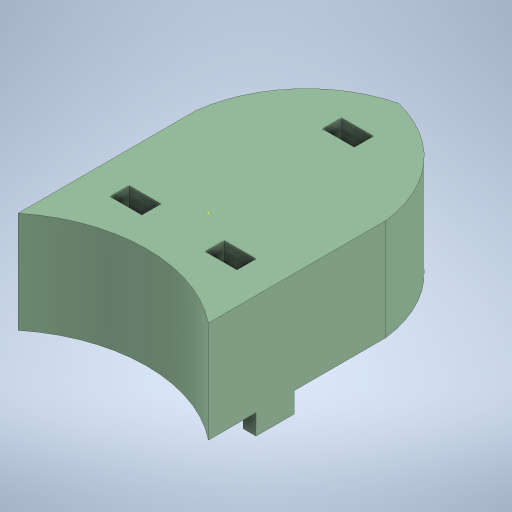
# Autodesk Inventor part: NORGATE
Saved by Autodesk Inventor 2024 (Build 280153000, 153)
## iProperties
Created: 2024-01-22
Part Number: NORGATE
Material: Generic
Document SubType Name: Modeling
Designer: Jetsan
Density: 1 g/cm^3
Appearance: Rubber - Green
Author: Jetsan
Autodesk Inventor part; units mm, degrees
ref_plane "YZ Plane" through (0, 0, 0) normal (1, 0, 0) x (0, 1, 0)
ref_plane "XZ Plane" through (0, 0, 0) normal (0, 1, 0) x (-1, 0, 0)
ref_plane "XY Plane" through (0, 0, 0) normal (0, 0, 1) x (1, 0, 0)
sketch "Sketch1" plane through (0, 0, 0) normal (0, 1, 0) x (-1, 0, 0)
  line L0 (-7.5, 7.5) -> (7.5, 7.5)
  line L1 (7.5, 7.5) -> (7.5, -7.5)
  line L2 (7.5, -7.5) -> (-7.5, -7.5)
  line L3 (-7.5, -7.5) -> (-7.5, 7.5)
  line L4 (-7.5, 7.5) -> (7.5, -7.5) construction
  line L5 (7.5, 7.5) -> (-7.5, -7.5) construction
  circle A0 centre (0, -7.5) radius 7.5 construction
  arc A1 (-7.5, -7.5) -> (7.5, -7.5) centre (0, -7.5) ccw
  arc A2 (0, -15) -> (7.5, -6.5) centre (-2.4276, -5.2991) ccw
  arc A3 (-7.5, -6.5) -> (0, -15) centre (2.4276, -5.2991) ccw
  point P0 (0, 0)
  dimension "d0" = 15
  dimension "d1" = 15
  dimension "d106" = 10
  dimension "d107" = 10
  dimension "d108" = 14
  dimension "d109" = 14
  constraints: 12 end point, 7 point on circle, 3 centre point, 3 midpoint, 2 parallel, 2 point on line, 1 coincident, 1 horizontal, 1 horizontal alignment, 1 perpendicular, 2 other
  measures "d0" distance of L0.end L1.end
  measures "d1" distance of L0.start L0.end
  measures "d106" radius of A2
  measures "d107" radius of A3
  measures "d108" distance from line of L0 A2.end
  measures "d109" distance from line of L0 A3.start
extrude "Extrusion1" add sketch "Sketch1" along normal blind 8 contours L0 L1 A2 L2 A3 L3 | L2 A2 A3
sketch "Sketch2" plane through (0, 0, 0) normal (0, -1, 0) x (1, 0, 0)
  line L0 (7.5, 11.25) -> (-7.5, 11.25)
  line L1 (-7.5, 11.25) -> (-7.5, -18.75)
  line L2 (-7.5, -18.75) -> (7.5, -18.75)
  line L3 (7.5, -18.75) -> (7.5, 11.25)
  line L4 (7.5, 11.25) -> (-7.5, -18.75) construction
  line L5 (-7.5, 11.25) -> (7.5, -18.75) construction
  line L6 (-7.5, 7.5) -> (7.5, 7.5) projected
  line L7 (7, 10.75) -> (-7, 10.75) construction
  line L8 (-7, 10.75) -> (-7, -18.25) construction
  line L9 (-7, -18.25) -> (7, -18.25) construction
  line L10 (7, -18.25) -> (7, 10.75) construction
  line L11 (7, 10.75) -> (-7, -18.25) construction
  line L12 (-7, 10.75) -> (7, -18.25) construction
  arc A0 (-7.5, 11.25) -> (7.5, 11.25) centre (0, 17.8644) ccw
  point P0 (0, 0)
  point P1 (0, -3.75)
  dimension "d4" = 15
  dimension "d5" = 30
  dimension "d6" = 3.75
  dimension "d18" = 0.5
  dimension "d19" = 0.5
  dimension "d99" = 10
  constraints: 24 end point, 4 midpoint, 4 parallel, 2 horizontal, 2 perpendicular, 2 point on circle, 1 centre point
  measures "d4" distance of L2.end L1.end
  measures "d5" distance of L1.end L0.end
  measures "d6" distance between parallel lines of L0 L6
  measures "d18" distance between parallel lines of L2 L9
  measures "d19" distance between parallel lines of L3 L10
  measures "d99" radius of A0
sketch "Sketch4" plane through (0, 0, 0) normal (0, -1, 0) x (1, 0, 0)
  line L0 (-7.5, -6.5) -> (-7.5, 7.5) projected
  line L1 (-7.5, 3.75) -> (-6.5, 3.75)
  line L2 (-6.5, 3.75) -> (-6.5, 0.75)
  line L3 (-6.5, 0.75) -> (-7.5, 0.75)
  line L4 (-7.5, 0.75) -> (-7.5, 3.75)
  line L5 (7.5, 7.5) -> (7.5, -6.5) projected
  line L6 (7.5, 0.75) -> (6.5, 0.75)
  line L7 (6.5, 0.75) -> (6.5, 3.75)
  line L8 (6.5, 3.75) -> (7.5, 3.75)
  line L9 (7.5, 3.75) -> (7.5, 0.75)
  line L10 (-7.5, -18.75) -> (7.5, -18.75) construction
  line L11 (7.5, -18.75) -> (7.5, 11.25) construction
  line L12 (7.5, 11.25) -> (-7.5, 11.25) construction
  line L13 (-7.5, 11.25) -> (-7.5, -18.75) construction
  line L14 (-7.5, -18.75) -> (7.5, 11.25) construction
  line L15 (7.5, -18.75) -> (-7.5, 11.25) construction
  line L16 (-7.5, 7.5) -> (7.5, 7.5) construction
  arc A0 (-7.5, -7.5) -> (7.5, -7.5) centre (0, -7.5) ccw construction
  point P0 (0, 0)
  point P1 (0, -3.75)
  point P2 (0, -15)
  point P3 (-7, 3.75)
  point P4 (7.5, 3.75)
  dimension "d20" = 1
  dimension "d21" = 3
  dimension "d22" = 1
  dimension "d23" = 3
  dimension "d24" = 15
  dimension "d25" = 30
  dimension "d26" = 3.75
  dimension "d27" = 3.75
  dimension "d28" = 7.5
  constraints: 28 end point, 6 parallel, 3 horizontal, 3 midpoint, 3 perpendicular, 3 point on line, 1 point on circle
  measures "d20" distance of L2.end L3.end
  measures "d21" distance of L1.end L2.end
  measures "d22" distance of L7.end L8.end
  measures "d23" distance of L6.end L7.end
  measures "d24" distance of L12.end L11.end
  measures "d25" distance of L11.end L10.end
  measures "d26" distance between parallel lines of L16 L12
  measures "d27" distance from line of L10 point (0, -15)
  measures "d28" distance from line of L12 point (-7, 3.75)
extrude "Extrusion3" add sketch "Sketch4" along normal blind 1.6
sketch "Sketch17" plane through (0, 0, 0) normal (0, -1, 0) x (1, 0, 0)
  line L0 (-7.5, 7.5) -> (7.5, 7.5) projected
  arc A0 (-7.5, 7.5) -> (7.5, 7.5) centre (0, 16.8675) ccw
  line L1 (7.5, 7.5) -> (-7.5, 7.5)
  point P0 (0, 0)
  dimension "d100" = 12
  constraints: 2 end point, 2 point on circle, 1 centre point, 1 horizontal
  measures "d100" radius of A0
extrude "Extrusion11" cut sketch "Sketch17" against normal blind 8
sketch "Sketch6" plane through (0, 0, 0) normal (0, -1, 0) x (1, 0, 0)
  line L0 (7.5, 11.25) -> (-7.5, 11.25)
  line L1 (-7.5, 11.25) -> (-7.5, -18.75)
  line L2 (-7.5, -18.75) -> (7.5, -18.75)
  line L3 (7.5, -18.75) -> (7.5, 11.25)
  line L4 (7.5, 11.25) -> (-7.5, -18.75) construction
  line L5 (-7.5, 11.25) -> (7.5, -18.75) construction
  line L6 (7, 10.75) -> (-7, 10.75) construction
  line L7 (-7, 10.75) -> (-7, -18.25) construction
  line L8 (-7, -18.25) -> (7, -18.25) construction
  line L9 (7, -18.25) -> (7, 10.75) construction
  line L10 (7, 10.75) -> (-7, -18.25) construction
  line L11 (-7, 10.75) -> (7, -18.25) construction
  circle A0 centre (0, -3.75) radius 1.25
  circle A1 centre (0, -3.75) radius 1.75
  line L12 (-6.5, 6.5) -> (6.5, 6.5)
  line L13 (6.5, 6.5) -> (6.5, -7.5)
  line L14 (6.5, -7.5) -> (-6.5, -7.5)
  line L15 (-6.5, -7.5) -> (-6.5, 6.5)
  line L16 (-7.5, 7.5) -> (7.5, 7.5) projected
  arc A2 (-7.5, -7.5) -> (7.5, -7.5) centre (0, -7.5) ccw projected
  circle A3 centre (0, -7.5) radius 6.5
  line L17 (0, 11.25) -> (0, -15) construction
  arc A4 (-6.5, 5.5) -> (6.5, 5.5) centre (0, 15.8675) ccw
  line L18 (6.5, 5.5) -> (-6.5, 5.5) construction
  line L19 (6.5, 5.5) -> (19.5, 5.5) construction
  arc A5 (-7.5, 7.5) -> (7.5, 7.5) centre (0, 16.8675) ccw projected
  point P0 (0, 0)
  point P1 (-7.5, -3.75)
  dimension "d31" = 15
  dimension "d32" = 30
  dimension "d34" = 0.5
  dimension "d35" = 0.5
  dimension "d36" = 2.5
  dimension "d37" = 0.5
  dimension "d38" = 1
  dimension "d39" = 1
  dimension "d40" = 1
  dimension "d41" = 1
  dimension "d103" = 180
  dimension "d104" = 1
  dimension "d105" = 1
  constraints: 38 end point, 6 midpoint, 6 parallel, 4 horizontal, 3 centre point, 3 coincident, 3 perpendicular, 3 point on circle, 2 point on line, 1 collinear, 3 other
  measures "d31" distance of L2.end L1.end
  measures "d32" distance of L1.end L0.end
  measures "d34" distance between parallel lines of L2 L8
  measures "d35" distance between parallel lines of L3 L9
  measures "d36" diameter of A0
  measures "d37" radial gap between concentric circles of A0 A1
  measures "d38" distance between parallel lines of L16 L12
  measures "d39" distance from line of point (-7.5, -3.75) L15
  measures "d40" distance between parallel lines of L3 L13
  measures "d103" angle of L18 L19
  measures "d104" distance of A5.centre A4.centre
  measures "d105" distance of L12.end L18.start
extrude "Extrusion4" cut sketch "Sketch6" against normal blind 2.5 contours L13 A3 L15 A4 | A3 L14 | L14 A3 | A0
sketch "Sketch10" plane through (0, 8, 0) normal (0, 1, 0) x (1, 0, 0)
  point P0 (0, 0)
sketch "Sketch11" plane through (0, 0, 0) normal (0, -1, 0) x (1, 0, 0)
  line L0 (-5, 2.75) -> (-2.5, 2.75)
  line L1 (-2.5, 2.75) -> (-2.5, 1.25)
  line L2 (-2.5, 1.25) -> (-5, 1.25)
  line L3 (-5, 1.25) -> (-5, 2.75)
  line L4 (2.5, 2.75) -> (5, 2.75)
  line L5 (5, 2.75) -> (5, 1.25)
  line L6 (5, 1.25) -> (2.5, 1.25)
  line L7 (2.5, 1.25) -> (2.5, 2.75)
  line L8 (-6.5, 3.75) -> (-7.5, 3.75) projected
  line L9 (-6.5, 0.75) -> (-6.5, 3.75) projected
  line L10 (6.5, 3.75) -> (6.5, 0.75) projected
  line L11 (-6.5, 6.5) -> (6.5, 6.5) projected
  line L12 (-1.25, -11.75) -> (1.25, -11.75)
  line L13 (1.25, -11.75) -> (1.25, -10.25)
  line L14 (1.25, -10.25) -> (-1.25, -10.25)
  line L15 (-1.25, -10.25) -> (-1.25, -11.75)
  point P0 (0, 0)
  point P1 (-3.75, 2.75)
  point P2 (3.75, 2.75)
  point P3 (1.25, -11)
  point P4 (2.5, 2)
  point P5 (0, -10.25)
  point P6 (3.75, 1.25)
  dimension "d51" = 2.5
  dimension "d52" = 1.5
  dimension "d53" = 1
  dimension "d55" = 2.75
  dimension "d56" = 2.75
  dimension "d57" = 3.75
  dimension "d60" = 13
  dimension "d61" = 3.75
  dimension "d62" = 3.75
  constraints: 24 end point, 6 midpoint, 6 parallel, 4 equal length, 3 horizontal, 3 perpendicular
  measures "d51" distance of L0.start L0.end
  measures "d52" distance of L0.end L1.end
  measures "d53" distance between parallel lines of L8 L0
  measures "d55" distance from line of L9 point (-3.75, 2.75)
  measures "d56" distance from line of L10 point (3.75, 2.75)
  measures "d57" distance between parallel lines of L11 L4
  measures "d60" vertical distance of point (1.25, -11) point (2.5, 2)
  measures "d61" horizontal distance of point (0, -10.25) point (3.75, 1.25)
  measures "d62" horizontal distance of point (0, -10.25) point (-3.75, 2.75)
extrude "Extrusion8" cut sketch "Sketch11" against normal blind 10
sketch "Sketch12" plane through (0, 2.5, 0) normal (0, -1, 0) x (1, 0, 0)
  line L0 (5, 1.25) -> (5, 2.75) construction
  line L1 (2.5, 1.25) -> (5, 1.25) construction
  line L2 (5, 2.75) -> (2.5, 2.75) construction
  line L3 (2.5, 2.75) -> (2.5, 1.25) construction
  line L4 (2.5, 1.25) -> (5, 1.25) construction
  line L5 (5, 1.25) -> (5, 2.75) construction
  line L6 (-2.5, 1.25) -> (-2.5, 2.75) construction
  line L7 (-2.5, 1.25) -> (-5, 1.25) construction
  line L8 (-2.5, 2.75) -> (-5, 2.75) construction
  line L9 (-5, 2.75) -> (-5, 1.25) construction
  line L10 (-5, 1.25) -> (-2.5, 1.25) construction
  line L11 (-2.5, 1.25) -> (-2.5, 2.75) construction
  line L12 (-1.25, -10.25) -> (1.25, -10.25) construction
  line L13 (-1.25, -10.25) -> (-1.25, -11.75) construction
  line L14 (1.25, -10.25) -> (-1.25, -10.25) construction
  line L15 (-1.25, -10.25) -> (-1.25, -11.75) construction
  line L16 (-1.25, -11.75) -> (1.25, -11.75) construction
  line L17 (1.25, -11.75) -> (1.25, -10.25) construction
  line L18 (5.5, 2.75) -> (2, 2.75)
  line L19 (2, 2.75) -> (2, 1.25)
  line L20 (2, 1.25) -> (5.5, 1.25)
  line L21 (5.5, 1.25) -> (5.5, 2.75)
  line L22 (1.75, -10.25) -> (-1.75, -10.25)
  line L23 (-1.75, -10.25) -> (-1.75, -11.75)
  line L24 (-1.75, -11.75) -> (1.75, -11.75)
  line L25 (1.75, -11.75) -> (1.75, -10.25)
  line L26 (-2, 2.75) -> (-5.5, 2.75)
  line L27 (-5.5, 2.75) -> (-5.5, 1.25)
  line L28 (-5.5, 1.25) -> (-2, 1.25)
  line L29 (-2, 1.25) -> (-2, 2.75)
  point P0 (0, 0)
  point P1 (-2.5, 2)
  point P2 (-2, 2)
  point P3 (-3.75, 1.25)
  point P4 (-3.75, 1.25)
  point P5 (-3.75, 2.75)
  point P6 (-3.75, 2.75)
  point P7 (-5, 2)
  point P8 (-5.5, 2)
  point P9 (1.25, -11)
  point P10 (1.75, -11)
  point P11 (0, -11.75)
  point P12 (-1.25, -11)
  dimension "d63" = 0.5
  dimension "d64" = 0
  dimension "d65" = 0
  dimension "d67" = 0.5
  dimension "d68" = 0
  dimension "d69" = 0
  dimension "d70" = 0.5
  dimension "d71" = 0.5
  dimension "d72" = 0
  dimension "d73" = 0
  dimension "d74" = 0.5
  dimension "d96" = 0.5
  constraints: 48 end point, 12 midpoint, 12 parallel, 6 horizontal, 6 perpendicular
  measures "d63" distance of point (-2.5, 2) point (-2, 2)
  measures "d64" distance of point (-3.75, 1.25) point (-3.75, 1.25)
  measures "d65" distance of point (-3.75, 2.75) point (-3.75, 2.75)
  measures "d67" distance of point (1.25, -11) point (1.75, -11)
  measures "d68" distance from line of L24 point (0, -11.75)
  measures "d69" distance between parallel lines of L22 L12
  measures "d70" distance from line of L23 point (-1.25, -11)
  measures "d71" distance between parallel lines of L0 L21
  measures "d72" distance between parallel lines of L20 L1
  measures "d73" distance between parallel lines of L18 L2
  measures "d74" distance between parallel lines of L19 L3
  measures "d96" distance between parallel lines of L27 L9
extrude "Extrusion9" cut sketch "Sketch12" against normal blind 1
sketch "Sketch16" plane through (0, 2.5, 0) normal (0, -1, 0) x (1, 0, 0)
  line L0 (-6.5, -7.5) -> (-6.5, 5.5) construction
  line L1 (-0.5, 4.8675) -> (0.5, 4.8675)
  line L2 (0.5, 4.8675) -> (0.5, -2.5)
  line L3 (0.5, -2.5) -> (-0.5, -2.5)
  line L4 (-0.5, -2.5) -> (-0.5, 4.8675)
  circle A0 centre (0, -3.75) radius 1.75 construction
  circle A1 centre (0, -3.75) radius 1.75 construction
  line L5 (-6.5, -2.5) -> (6.5174, -2.5) construction
  circle A2 centre (0, -3.75) radius 1.75 construction
  circle A3 centre (0, -3.75) radius 1.25 construction
  line L6 (6.5, 0.75) -> (6.5, -7.5) projected
  line L7 (-6.5, -5.873) -> (6.5, -5.873)
  line L8 (6.5, -5.873) -> (6.5, -6.873)
  line L9 (6.5, -6.873) -> (-6.5, -6.873)
  line L10 (-6.5, -6.873) -> (-6.5, -5.873)
  arc A4 (-7.5, 7.5) -> (7.5, 7.5) centre (0, 16.8675) ccw projected
  point P0 (0, 0)
  point P1 (-6.5, 6.5)
  point P2 (6.5, 6.5)
  point P3 (0, 4.8675)
  point P4 (0.0087, -2.5)
  dimension "d94" = 1
  dimension "d95" = 1
  constraints: 18 end point, 4 parallel, 4 point on line, 3 perpendicular, 2 horizontal, 2 midpoint, 1 centre point, 1 coincident, 1 point on circle, 1 tangent
  measures "d94" distance between parallel lines of L2 L4
  measures "d95" distance between parallel lines of L9 L7
extrude "Extrusion10" add sketch "Sketch16" along normal blind 2.5 contours L1 L2 L3 L4
sketch "Sketch14" plane through (0, 2.5, 0) normal (0, -1, 0) x (1, 0, 0)
  line L0 (5, 2.75) -> (2.5, 2.75) construction
  line L1 (2.5, 2.75) -> (2.5, 1.25) construction
  line L2 (2.5, 1.25) -> (5, 1.25) construction
  line L3 (5, 1.25) -> (5, 2.75) construction
  line L4 (5.5, 3.25) -> (2, 3.25)
  line L5 (2, 3.25) -> (2, 0.75)
  line L6 (2, 0.75) -> (5.5, 0.75)
  line L7 (5.5, 0.75) -> (5.5, 3.25)
  dimension "d86" = 0.5
  dimension "d87" = 0.5
  constraints: 16 end point, 4 parallel, 2 horizontal, 2 perpendicular
  measures "d86" distance between parallel lines of L4 L0
  measures "d87" distance between parallel lines of L5 L1
sketch "Sketch15" plane through (0, 3.5, 0) normal (0, -1, 0) x (1, 0, 0)
  line L0 (5, 2.75) -> (2.5, 2.75)
  line L1 (2.5, 2.75) -> (2.5, 1.25)
  line L2 (2.5, 1.25) -> (5, 1.25)
  line L3 (5, 1.25) -> (5, 2.75)
  point P0 (0, 0)
  constraints: 8 end point, 2 parallel, 1 horizontal, 1 perpendicular
sketch "Sketch8" plane through (0, 0, -3.75) normal (0, -1, 0) x (1, 0, 0)
  circle A0 centre (0, 0) radius 1.75
  circle A1 centre (0, 0) radius 1.75 projected
  circle A2 centre (0, 0) radius 1.5
  point P0 (0, 3.75)
  dimension "d46" = 0.25
  constraints: 2 centre point, 2 coincident, 1 concentric
  measures "d46" radial gap between concentric circles of A2 A0
sketch "Sketch7" plane through (0, 2.5, -3.75) normal (0, -1, 0) x (1, 0, 0)
  circle A0 centre (0, 0) radius 1.25
  point P0 (0, 3.75)
  constraints: 1 centre point
body "Solid1"
